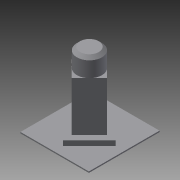
# Autodesk Inventor part: BUTTON
Saved by Autodesk Inventor 2014 SP1 (Build 180222100, 222)
## iProperties
Created: 2013-12-02
Part Number: BUTTON
Material: Generic
Document SubType Name: Modeling
Designer: Dominik
Density: 1 g/cm^3
Appearance: Default
Author: Dominik
Autodesk Inventor part; units mm, degrees
ref_plane "YZ Plane" through (0, 0, 0) normal (1, 0, 0) x (0, 1, 0)
ref_plane "XZ Plane" through (0, 0, 0) normal (0, 1, 0) x (-1, 0, 0)
ref_plane "XY Plane" through (0, 0, 0) normal (0, 0, 1) x (1, 0, 0)
sketch "Sketch3" plane through (0, 0, 0) normal (0, 0, 1) x (1, 0, 0)
  line L0 (0, 0) -> (6, 0) construction
  line L1 (6, 0) -> (6, 6) construction
  line L2 (6, 6) -> (0, 6) construction
  line L3 (0, 6) -> (0, 0) construction
  line L4 (0, 0) -> (6, 6) construction
  line L5 (0, 6) -> (6, 0) construction
  line L6 (3, 6) -> (3, 0) construction
  line L7 (6, 3) -> (0, 3) construction
  line L8 (3, 6) -> (6, 3) construction
  line L9 (6, 3) -> (3, 0) construction
  line L10 (3, 0) -> (0, 3) construction
  line L11 (0, 3) -> (3, 6) construction
  line L12 (3, 5.8586) -> (0.1414, 3)
  line L13 (0.1414, 3) -> (3, 0.1414)
  line L14 (3, 0.1414) -> (5.8586, 3)
  line L15 (3, 5.8586) -> (5.8586, 3)
  dimension "d9" = 6
  dimension "d10" = 6
  dimension "d11" = 0.1
  dimension "d12" = 0.1
  constraints: 32 end point, 4 midpoint, 2 point on line, 1 parallel
  measures "d9" distance between parallel lines of L1 L3
  measures "d10" distance between parallel lines of L2 L0
  measures "d11" distance between parallel lines of L11 L12
  measures "d12" distance between parallel lines of L8 L15
extrude "Extrusion3" add sketch "Sketch3" along normal blind 8
sketch "Sketch4" plane through (0, 0, 8) normal (0, 0, 1) x (1, 0, 0)
  line L0 (0.1414, 3) -> (5.8586, 3) construction
  line L1 (3, 0.1414) -> (3, 5.8586) construction
  circle A0 centre (3, 3) radius 2.0213
  point P0 (0, 0)
  constraints: 4 end point, 1 centre point, 1 midpoint
extrude "Extrusion4" add sketch "Sketch4" along normal blind 3
chamfer "Chamfer2" distance 0.5 angle 45 1 edges at (0.9787, 3, 11)
sketch "Sketch5" plane through (0, 0, 0) normal (0, 0, -1) x (-1, 0, 0)
  line L0 (-3, 5.8586) -> (-0.1414, 3) projected
  line L1 (-5.8586, 3) -> (-3, 5.8586) projected
  line L2 (-3, 0.1414) -> (-5.8586, 3) projected
  line L3 (-0.1414, 3) -> (-3, 0.1414) projected
  line L4 (1.2728, 3) -> (-3, 7.2728)
  line L5 (-3, 7.2728) -> (-7.2728, 3)
  line L6 (-7.2728, 3) -> (-3, -1.2728)
  line L7 (-3, -1.2728) -> (1.2728, 3)
  point P0 (0, 0)
  dimension "d20" = 1
  constraints: 8 end point, 3 other
  measures "d20" distance between parallel lines of L0 L4
extrude "Extrusion5" add sketch "Sketch5" along normal blind 1 contours L0 L3 L2 L1 | L7 L6 L5 L4
sketch "Sketch6" plane through (0, 0, -1) normal (0, 0, -1) x (-1, 0, 0)
  line L0 (1.2728, 3) -> (-3, 7.2728) projected
  line L1 (-3, 7.2728) -> (-7.2728, 3) projected
  line L2 (-7.2728, 3) -> (-3, -1.2728) projected
  line L3 (-3, -1.2728) -> (1.2728, 3) projected
  line L4 (-8.684, 8.684) -> (2.4119, 8.684)
  line L5 (2.4119, 8.684) -> (2.4119, -2.7747)
  line L6 (2.4119, -2.7747) -> (-8.684, -2.7747)
  line L7 (-8.684, -2.7747) -> (-8.684, 8.684)
  point P0 (0, 0)
  constraints: 8 end point
extrude "printing support" add sketch "Sketch6" against normal blind 0.2
equation "\"d12\" = d11"
body "Solid2"
